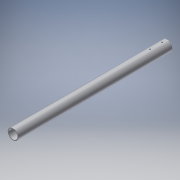
# Autodesk Inventor part: 2f2barm
Saved by Autodesk Inventor 2016 (Build 200138000, 138)
## iProperties
Company: HERA Project
Created: 2013-07-11
Part Number: 2f2barm
Material: PVC-Piping
Description: PVC arm for feed backplane
Document SubType Name: Modeling
Designer: David DeBoer
Mass: 174.937 g
Surface Area: 877.469 cm^2
Volume: 124.955 cm^3
Density: 1.4 g/cm^3
Appearance: Smooth - White
Title: feed-bppvcarm
Author: David DeBoer
Autodesk Inventor part; units mm, degrees
ref_plane "YZ Plane" through (0, 0, 0) normal (1, 0, 0) x (0, 1, 0)
ref_plane "XZ Plane" through (0, 0, 0) normal (0, 1, 0) x (-1, 0, 0)
ref_plane "XY Plane" through (0, 0, 0) normal (0, 0, 1) x (1, 0, 0)
sketch "Sketch1" plane through (0, 0, 0) normal (0, 0, 1) x (1, 0, 0)
  circle A0 centre (0, 0) radius 11
  circle A1 centre (0, 0) radius 9.38
  dimension "d0" = 22
  dimension "d2" = 1.62
  constraints: 2 centre point, 1 coincident
  measures "d0" diameter of A0
  measures "d2" radial gap between concentric circles of A1 A0
extrude "Extrusion1" add sketch "Sketch1" along normal blind 320
sketch "Sketch6" plane through (0, 0, 320) normal (0, 0, 1) x (1, 0, 0)
  circle A0 centre (0, 0) radius 9.38 projected
  circle A1 centre (0, 0) radius 11 projected
  line L0 (-3.2787, 10.5) -> (3.2787, 10.5)
  dimension "d18" = 10.5
  constraints: 2 end point, 2 point on circle, 1 horizontal
  measures "d18" distance from line of A0.centre L0
extrude "Extrusion3" cut sketch "Sketch6" against normal through all contours L0 A1 picked at (-0.3693, 10.648)
sketch "Sketch8" plane through (-3.2787, 10.5, 320) normal (0, 1, 0) x (1, 0, 0)
  circle A0 centre (3.2787, 310) radius 1.7934
  point P0 (3.2787, 320)
  dimension "d47" = 10
  constraints: 1 centre point
  measures "d47" distance of A0.centre point (3.279, 320)
hole "Hole4" at (0, 10.5, 10) direction (0, -1, 0) diameter 3 depth 8 tip angle 118
sketch "Sketch9" plane through (-3.2787, 10.5, 320) normal (0, 1, 0) x (1, 0, 0)
  circle A0 centre (3.2787, 310) radius 1.5 projected
  circle A1 centre (3.2787, 285) radius 1.2403
  point P0 (3.2787, 320)
  dimension "d55" = 25
  constraints: 1 centre point
  measures "d55" distance of A1.centre A0.centre
hole "Hole5" at (0, 10.5, 35) direction (0, -1, 0) diameter 3 depth 8 tip angle 118
body "Solid1"
